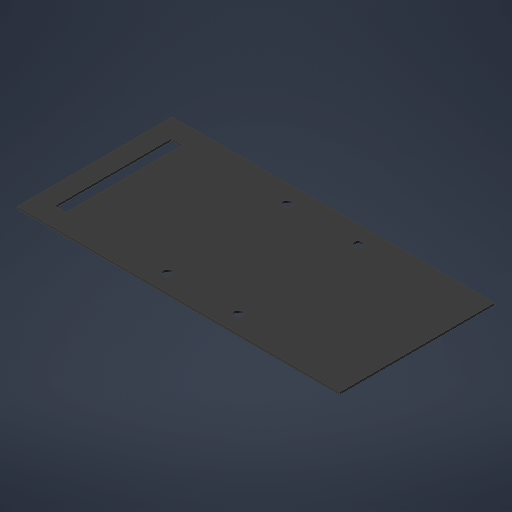
# Autodesk Inventor part: CoverImpresoraTermica
Saved by Autodesk Inventor 2026.1 (Build 301233020, 233B)
## iProperties
Created: 2025-11-04
Part Number: CoverImpresoraTermica
Material: Generic
Document SubType Name: Modeling
Designer: Tito Luyo Murata
Density: 1 g/cm^3
Appearance: Default
Author: Tito Luyo Murata
Autodesk Inventor part; units mm, degrees
ref_plane "YZ Plane" through (0, 0, 0) normal (1, 0, 0) x (0, 1, 0)
ref_plane "XZ Plane" through (0, 0, 0) normal (0, 1, 0) x (-1, 0, 0)
ref_plane "XY Plane" through (0, 0, 0) normal (0, 0, 1) x (1, 0, 0)
sketch "Sketch1" plane through (0, 0, 0) normal (0, 1, 0) x (-1, 0, 0)
  line L0 (0, 0) -> (250, 0)
  line L1 (250, 0) -> (250, -120)
  line L2 (250, -120) -> (0, -120)
  line L3 (0, -120) -> (0, 0)
  circle A0 centre (92, -13.5) radius 3.5
  circle A1 centre (92, -106.5) radius 3.5
  circle A2 centre (147, -13.5) radius 3.5
  circle A3 centre (147, -106.5) radius 3.5
  line L4 (236, -14.5) -> (227, -14.5)
  line L5 (227, -14.5) -> (227, -105.5)
  line L6 (227, -105.5) -> (236, -105.5)
  line L7 (236, -105.5) -> (236, -14.5)
  point P0 (0, -60)
  point P1 (250, -60)
  dimension "d0" = 250
  dimension "d1" = 120
  dimension "d2" = 7
  dimension "d3" = 92
  dimension "d4" = 7
  dimension "d5" = 92
  dimension "d6" = 93
  dimension "d7" = 46.5
  dimension "d8" = 7
  dimension "d9" = 7
  dimension "d10" = 55
  dimension "d11" = 93
  dimension "d12" = 55
  dimension "d13" = 46.5
  dimension "d14" = 9
  dimension "d15" = 91
  dimension "d16" = 45.5
  dimension "d17" = 80
  constraints: 16 end point, 4 centre point, 4 parallel, 2 horizontal, 2 midpoint, 2 perpendicular
  measures "d0" distance of L1.end L2.end
  measures "d1" distance of L0.end L1.end
  measures "d2" diameter of A0
  measures "d3" distance from line of L3 A0.centre
  measures "d4" diameter of A1
  measures "d5" distance from line of L3 A1.centre
  measures "d6" distance of A1.centre A0.centre
  measures "d7" vertical distance of point (0, -60) A0.centre
  measures "d8" diameter of A2
  measures "d9" diameter of A3
  measures "d10" distance of A0.centre A2.centre
  measures "d11" distance of A3.centre A2.centre
  measures "d12" distance of A1.centre A3.centre
  measures "d13" vertical distance of point (0, -60) A2.centre
  measures "d14" distance between parallel lines of L5 L7
  measures "d15" distance between parallel lines of L6 L4
  measures "d16" distance from line of point (250, -60) L4
  measures "d17" distance from line of A2.centre L5
extrude "Extrusion1" add sketch "Sketch1" along normal blind 2
equation "\"d2\" = hueco_diam"
equation "\"d3\" = primer_hueco_dist"
equation "\"d4\" = hueco_diam"
equation "\"d5\" = primer_hueco_dist"
equation "\"d6\" = huecos_horiz_dist"
equation "\"d7\" = 0.5 * huecos_horiz_dist"
equation "\"d8\" = hueco_diam"
equation "\"d9\" = hueco_diam"
equation "\"d11\" = huecos_horiz_dist"
equation "\"d13\" = 0.5 * huecos_horiz_dist"
equation "\"hueco_diam\" = 7"
equation "\"primer_hueco_dist\" = 92"
equation "\"huecos_horiz_dist\" = 93"
body "Solid1"
